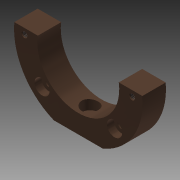
# Autodesk Inventor part: Mount
Saved by Autodesk Inventor 2014 (Build 180170000, 170)
## iProperties
Created: 2014-11-07
Part Number: Mount
Material: Bronze, Soft Tin
Document SubType Name: Modeling
Designer: nfitch
Mass: 59.769 g
Surface Area: 35.9496 cm^2
Volume: 6.73529 cm^3
Density: 8.874 g/cm^3
Appearance: Bronze - Satin
Author: nfitch
Autodesk Inventor part; units mm, degrees
ref_plane "YZ Plane" through (0, 0, 0) normal (1, 0, 0) x (0, 1, 0)
ref_plane "XZ Plane" through (0, 0, 0) normal (0, 1, 0) x (-1, 0, 0)
sketch "Sketch2" plane through (0, 0, 0) normal (0, 0, 1) x (1, 0, 0)
  circle A0 centre (0, 0) radius 27.5
  dimension "d44" = 55
  constraints: 1 centre point
  measures "d44" diameter of A0
extrude "Extrusion1" add sketch "Sketch2" along normal blind 10
sketch "Sketch4" plane through (0, 0, 10) normal (0, 0, 1) x (1, 0, 0)
  point P0 (0, 0)
  point P1 (-15.5, -15.5)
  point P2 (15.5, -15.5)
hole "Hole1" at (-15.5, -15.5, 10) at (15.5, -15.5, 10) direction (0, 0, -1) diameter 3.4 end through all counterbore diameter 6.5 counterbore depth 3 clearance for "Socket Head Cap Screw" size "M3" standard "Ansi Metric M Profile"
sketch "Sketch7" plane through (0, 0, 10) normal (0, 0, 1) x (1, 0, 0)
  circle A0 centre (0, 0) radius 17.5
  dimension "d26" = 35
  constraints: 1 centre point
  measures "d26" diameter of A0
extrude "Extrusion4" cut sketch "Sketch7" against normal through all
sketch "Sketch8" plane through (0, 0, 10) normal (0, 0, 1) x (1, 0, 0)
  point P0 (-23.0125, 0)
  point P1 (23.0125, 0)
hole "Hole3" at (-23.0125, 0, 10) at (23.0125, 0, 10) direction (0, 0, -1) diameter 2.013 end through all thread size "M2.5x0.45" class "6H" standard "ANSI Metric M Profile"
chamfer "Chamfer1" distance 0.25 angle 45 1 edges at (-23.0125, 1.0065, 10)
chamfer "Chamfer2" distance 0.25 angle 45 1 edges at (23.0125, 1.0065, 10)
sketch "Sketch10" plane through (0, 0, 10) normal (0, 0, 1) x (1, 0, 0)
  line L0 (-15.5, -29.5673) -> (15.5, -29.5673)
  line L1 (15.5, -29.5673) -> (15.5, -25.4327)
  line L2 (15.5, -25.4327) -> (-15.5, -25.4327)
  line L3 (-15.5, -25.4327) -> (-15.5, -29.5673)
  line L4 (-15.5, -29.5673) -> (15.5, -25.4327) construction
  line L5 (15.5, -29.5673) -> (-15.5, -25.4327) construction
  line L6 (-30, 2.5) -> (30, 2.5)
  line L7 (30, 2.5) -> (30, 32.5)
  line L8 (30, 32.5) -> (-30, 32.5)
  line L9 (-30, 32.5) -> (-30, 2.5)
  point P0 (0, -27.5)
  dimension "d63" = 60
  dimension "d64" = 30
  constraints: 20 end point, 4 parallel, 2 horizontal, 2 midpoint, 2 perpendicular
  measures "d63" distance of L8.end L7.end
  measures "d64" distance of L7.end L6.end
extrude "Extrusion6" cut sketch "Sketch10" against normal through all
ref_plane "Work Plane1" through (-10.4608, -15.4327, 10) normal (0, -1, 0) x (1, 0, 0)
sketch "Sketch13" plane through (-10.4608, -15.4327, 10) normal (0, -1, 0) x (1, 0, 0)
  point P0 (10.4608, -10)
  point P1 (10.4608, -5)
hole "Hole5" at (0, -15.4327, 5) direction (0, -1, 0) diameter 4.5 end through all clearance for "Hex Head Machine Screw" size "M4" standard "Ansi Metric M Profile"
sketch "Sketch14" plane through (-10.4608, -15.4327, 10) normal (0, -1, 0) x (1, 0, 0)
  circle A0 centre (10.4608, -5) radius 3.5
  point P0 (10.4608, -10)
  dimension "d73" = 7
  constraints: 1 centre point
  measures "d73" diameter of A0
extrude "Extrusion7" cut sketch "Sketch14" along normal blind 6
body "Solid1"
